Autodesk Fusion 360 part; units mm, degrees
note: some values were not read from the file. Set by a fixed rule: which sketch regions a step uses.
(part 2 of 2)
sketch "Sketch27" plane through (0, 0, 2) normal (0, 0, 1) x (-1, 0, 0)
  line L0 (0, 6.5) -> (-2, 6.5)
  line L1 (-2, 6.5) -> (-2, 28)
  line L2 (-2, 28) -> (0, 28)
  line L3 (0, 28) -> (0, 6.5)
  circle A0 centre (-17.5, -19.5) radius 3
  line L4 (31.1094, 25.8906) -> (31.1094, 22.8906)
  line L5 (31.1094, 22.8906) -> (27.1094, 22.8906)
  line L6 (27.1094, 22.8906) -> (27.1094, 30.8906)
  line L7 (27.1094, 30.8906) -> (35.1094, 30.8906)
  line L8 (35.1094, 30.8906) -> (35.1094, 26.8906)
  line L9 (35.1094, 26.8906) -> (32.1094, 26.8906)
  arc A1 (32.1094, 26.8906) -> (31.1094, 25.8906) centre (32.1094, 25.8906) ccw
  circle A2 centre (13.9294, 15) radius 3
  circle A3 centre (13.9294, -15) radius 3
  circle A4 centre (21.9294, -25) radius 3
  circle A5 centre (5.9294, -25) radius 3
  line L10 (-68, -12) -> (-62, -12)
  line L11 (-62, -12) -> (-62, -33)
  line L12 (-62, -33) -> (62, -33)
  line L13 (62, -33) -> (62, -29)
  arc A6 (64, -27) -> (62, -29) centre (64, -29) ccw
  line L14 (64, -27) -> (68, -27)
  line L15 (68, -27) -> (68, 27)
  line L16 (68, 27) -> (53, 27)
  line L17 (53, 27) -> (53, 28)
  line L18 (53, 28) -> (62.2679, 28)
  arc A7 (62, 29) -> (62.2679, 28) centre (64, 29) ccw
  line L19 (62, 29) -> (62, 33)
  line L20 (62, 33) -> (-62, 33)
  line L21 (-62, 33) -> (-62, 2)
  line L22 (-62, 2) -> (-68, 2)
  line L23 (-68, 2) -> (-68, 1.5)
  line L24 (-68, 1.5) -> (-45, 1.5)
  line L25 (-45, 1.5) -> (-45, 0.5)
  line L26 (-45, 0.5) -> (-68, 0.5)
  line L27 (-68, 0.5) -> (-68, -12)
  circle A8 centre (5.9294, 25) radius 3
  circle A9 centre (21.9294, 25) radius 3
  circle A10 centre (-49.5, -19.5) radius 3
  circle A11 centre (58, -29) radius 3
  line L28 (13.9294, 15) -> (13.9294, -15) construction
  line L29 (26.4294, 11) -> (1.4294, 11)
  line L30 (1.4294, 11) -> (1.4294, -11)
  line L31 (1.4294, -11) -> (26.4294, -11)
  line L32 (26.4294, -11) -> (26.4294, 11)
  line L33 (26.4294, 11) -> (1.4294, -11) construction
  line L34 (1.4294, 11) -> (26.4294, -11) construction
  line L35 (1.4294, 11) -> (9.4294, 11)
  line L36 (9.4294, 11) -> (9.4294, 20)
  line L37 (9.4294, 20) -> (1.4294, 20)
  line L38 (1.4294, 20) -> (1.4294, 11)
  line L39 (26.4294, 11) -> (18.4294, 11)
  line L40 (18.4294, 11) -> (18.4294, 20)
  line L41 (18.4294, 20) -> (26.4294, 20)
  line L42 (26.4294, 20) -> (26.4294, 11)
  line L43 (1.4294, -11) -> (9.4294, -11)
  line L44 (9.4294, -11) -> (9.4294, -20)
  line L45 (9.4294, -20) -> (1.4294, -20)
  line L46 (1.4294, -20) -> (1.4294, -11)
  line L47 (26.4294, -11) -> (18.4294, -11)
  line L48 (18.4294, -11) -> (18.4294, -20)
  line L49 (18.4294, -20) -> (26.4294, -20)
  line L50 (26.4294, -20) -> (26.4294, -11)
  line L51 (1.4294, 0) -> (-12.5706, 0)
  line L52 (-12.5706, 0) -> (-12.5706, -30)
  line L53 (-12.5706, -30) -> (1.4294, -30)
  line L54 (1.4294, -30) -> (1.4294, 0)
  line L55 (-12.5706, 0) -> (-62.5706, 0)
  line L56 (-62.5706, 0) -> (-62.5706, -10)
  line L57 (-62.5706, -10) -> (-12.5706, -10)
  line L58 (-12.5706, -10) -> (-12.5706, 0)
  line L59 (-60.5706, 0) -> (-60.5706, -10)
  line L60 (-56.5706, 0) -> (-56.5706, -10)
  line L61 (-58.5706, 0) -> (-58.5706, -10)
  line L62 (-52.5706, 0) -> (-52.5706, -10)
  line L63 (-54.5706, 0) -> (-54.5706, -10)
  line L64 (-48.5706, 0) -> (-48.5706, -10)
  line L65 (-50.5706, 0) -> (-50.5706, -10)
  line L66 (-44.5706, 0) -> (-44.5706, -10)
  line L67 (-46.5706, 0) -> (-46.5706, -10)
  line L68 (-40.5706, 0) -> (-40.5706, -10)
  line L69 (-42.5706, 0) -> (-42.5706, -10)
  line L70 (-36.5706, 0) -> (-36.5706, -10)
  line L71 (-38.5706, 0) -> (-38.5706, -10)
  line L72 (-32.5706, 0) -> (-32.5706, -10)
  line L73 (-34.5706, 0) -> (-34.5706, -10)
  line L74 (-28.5706, 0) -> (-28.5706, -10)
  line L75 (-30.5706, 0) -> (-30.5706, -10)
  line L76 (-24.5706, 0) -> (-24.5706, -10)
  line L77 (-26.5706, 0) -> (-26.5706, -10)
  line L78 (-20.5706, 0) -> (-20.5706, -10)
  line L79 (-22.5706, 0) -> (-22.5706, -10)
  line L80 (-16.5706, 0) -> (-16.5706, -10)
  line L81 (-18.5706, 0) -> (-18.5706, -10)
  line L82 (-12.5706, 0) -> (-12.5706, -10)
  line L83 (-14.5706, 0) -> (-14.5706, -10)
  line L84 (-10.5706, 0) -> (-10.5706, -30)
  line L85 (-6.5706, 0) -> (-6.5706, -30)
  line L86 (-8.5706, 0) -> (-8.5706, -30)
  line L87 (-2.5706, 0) -> (-2.5706, -30)
  line L88 (-4.5706, 0) -> (-4.5706, -30)
  line L89 (1.4294, 0) -> (1.4294, -30)
  line L90 (-0.5706, 0) -> (-0.5706, -30)
  line L91 (3.4294, 20) -> (3.4294, -20)
  line L92 (4.4294, 11) -> (4.4294, -11)
  line L93 (6.4294, 20) -> (6.4294, -20)
  line L94 (4.4294, 20) -> (4.4294, 11)
  line L95 (4.4294, -30) -> (4.4294, 0)
  line L96 (7.4294, 11) -> (7.4294, -11)
  line L97 (9.4294, 20) -> (9.4294, -20)
  line L98 (7.4294, 20) -> (7.4294, 11)
  line L99 (7.4294, -30) -> (7.4294, 0)
  line L100 (24.4294, 20) -> (24.4294, -20)
  line L101 (23.4294, 20) -> (23.4294, 11)
  line L102 (21.4294, 20) -> (21.4294, -20)
  line L103 (23.4294, -11) -> (23.4294, 11)
  line L104 (23.4294, -20) -> (23.4294, -11)
  line L105 (20.4294, 20) -> (20.4294, 11)
  line L106 (18.4294, 20) -> (18.4294, -20)
  line L107 (20.4294, -11) -> (20.4294, 11)
  line L108 (20.4294, -20) -> (20.4294, -11)
  line L109 (16.4294, 11) -> (16.4294, -11)
  line L110 (15.4294, 11) -> (15.4294, -11)
  line L111 (14.4294, 11) -> (14.4294, -11)
  line L112 (13.4294, 11) -> (13.4294, -11)
  line L113 (12.4294, 11) -> (12.4294, -11)
  line L114 (11.4294, 11) -> (11.4294, -11)
  point P0 (13.9294, 0)
  dimension "d231" = 25
  dimension "d232" = 22
  dimension "d233" = 8
  dimension "d234" = 9
  dimension "d235" = 8
  dimension "d236" = 9
  dimension "d237" = 8
  dimension "d238" = 9
  dimension "d239" = 8
  dimension "d240" = 9
  dimension "d241" = 14
  dimension "d242" = 30
  dimension "d243" = 50
  dimension "d244" = 2
  dimension "d247" = 48
  dimension "d248" = 0
  dimension "d249" = 2
  dimension "d252" = 12
  dimension "d253" = 0
  dimension "d254" = 2
  dimension "d257" = 6
  dimension "d258" = 0
  dimension "d259" = 2
  dimension "d262" = -6
  dimension "d263" = 0
  dimension "d264" = 2
  dimension "d265" = 1
  dimension "d268" = -4
  dimension "d269" = 0
  constraint coincident A2.centre L28.start
  constraint coincident A3.centre L28.end
  constraint horizontal L29
  constraint perpendicular L29 L30
  constraint parallel L29 L31
  constraint parallel L30 L32
  constraint coincident L33 P0
  constraint coincident L34 P0
  constraint midpoint L28 P0
  constraint horizontal L35
  constraint vertical L36
  constraint horizontal L37
  constraint vertical L38
  constraint horizontal L39
  constraint vertical L40
  constraint horizontal L41
  constraint vertical L42
  constraint horizontal L43
  constraint vertical L44
  constraint horizontal L45
  constraint vertical L46
  constraint horizontal L47
  constraint vertical L48
  constraint horizontal L49
  constraint vertical L50
  constraint horizontal L51
  constraint vertical L52
  constraint horizontal L53
  constraint vertical L54
  constraint midpoint L30 L51.start
  constraint horizontal L55
  constraint vertical L56
  constraint horizontal L57
  constraint vertical L58
  constraint coincident L55 L59.start
  constraint coincident L57 L59.end
  constraint perpendicular L57 L59
  constraint coincident L51 L84.start
  constraint coincident L53 L84.end
  constraint perpendicular L53 L84
  constraint coincident L37 L91.start
  constraint coincident L45 L91.end
  constraint perpendicular L45 L91
  constraint coincident L41 L100.start
  constraint coincident L49 L100.end
  constraint perpendicular L49 L100
  constraint coincident L29 L109.start
  constraint coincident L31 L109.end
  constraint perpendicular L31 L109
  constraint coincident L29 L110.start
  constraint perpendicular L29 L110
  measures "d231" distance of L30.end L31.end
  measures "d232" distance of L29.end L30.end
  measures "d233" distance of L29.end L35.end
  measures "d234" distance of L29.end L37.end
  measures "d235" distance of L29.start L39.end
  measures "d236" distance of L29.start L41.end
  measures "d237" distance of L30.end L43.end
  measures "d238" distance of L30.end L45.end
  measures "d239" distance of L31.end L47.end
  measures "d240" distance of L31.end L49.end
  measures "d241" distance of L51.start L51.end
  measures "d242" distance of L51.start L53.end
  measures "d243" distance of L51.end L55.end
  measures "d244" distance of L56 L59
  measures "d249" distance of L52 L84
  measures "d254" distance of L89 L91
  measures "d259" distance of L32 L100
  measures "d264" distance of L106 L109
  measures "d265" distance of L109 L110
extrude "Extrude26" cut sketch "Sketch27" against normal blind 2 contours L31 L43 L44 L45 L97 L99 | L31 L43 L45 L93 L95 | L29 L31 L35 L43 L96 L97 L99 | L31 L43 L45 L46 L54 L89 L91 | L29 L31 L35 L43 L92 L93 L95 | L29 L30 L31 L35 L43 L54 L89 L91 | L29 L31 L113 L114 | L29 L35 L36 L37 L97 L98 | L29 L35 L37 L93 L94 | L29 L35 L37 L38 L91 | L29 L31 L112 L113 | L51 L53 L87 L90 | L29 L31 L110 L111 | L51 L53 L85 L88 | L29 L31 L109 L110 | L51 L53 L84 L86 | L29 L31 L39 L47 L106 L107 | L31 L47 L48 L49 L106 L108 | L29 L39 L40 L41 L105 L106 | L29 L31 L39 L47 L102 L103 | L31 L47 L49 L102 L104 | L52 L55 L57 L58 L82 L83 | L29 L39 L41 L101 L102 | L29 L31 L32 L39 L47 L100 | L31 L47 L49 L50 L100 | L55 L57 L80 L81 | L29 L39 L41 L42 L100 | L55 L57 L78 L79 | L55 L57 L76 L77 | L55 L57 L74 L75 | L55 L57 L72 L73 | L55 L57 L70 L71 | L55 L57 L68 L69 | L55 L57 L66 L67 | L55 L57 L64 L65 | L55 L57 L62 L63 | L55 L57 L60 L61 | L55 L56 L57 L59 bodies 1
